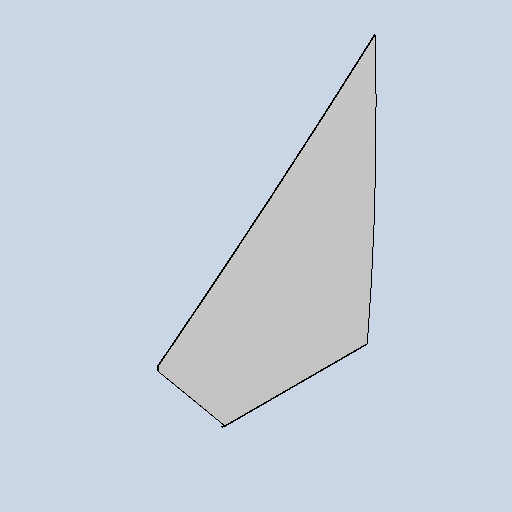
# Autodesk Inventor part: MSC 311 sheet left board face
Saved by Autodesk Inventor 2025 (Build 290162010, 162A)
## iProperties
Created: 2024-04-18
Part Number: MSC 311 sheet left board face
Material: AISI304
Document SubType Name: Sheet Metal
Designer: admin
Stock Number: МОО 311 лист левый борт морда
Mass: 48027.3 g
Surface Area: 40202.8 cm^2
Volume: 6003.41 cm^3
Density: 8 g/cm^3
Sheet Metal Rule: Default_mm
Sheet Metal Width: 980,000 mm
Sheet Metal Length: 1340,712 mm
Sheet Metal Area: 1313897,739 mm^2
Appearance: Default
Flat Pattern Width: 98 cm
Flat Pattern Length: 134.071 cm
Flat Pattern Area: 13139 cm^2
Author: admin
Autodesk Inventor part; units mm, degrees
ref_plane "YZ Plane" through (0, 0, 0) normal (1, 0, 0) x (0, 1, 0)
ref_plane "XZ Plane" through (0, 0, 0) normal (0, 1, 0) x (-1, 0, 0)
ref_plane "XY Plane" through (0, 0, 0) normal (0, 0, 1) x (1, 0, 0)
sketch "Sketch1" plane through (0, 0, 0) normal (0, 0, 1) x (1, 0, 0)
  line L0 (394.757121, -1035.809004) -> (394.757121, -1085.809004) construction
  line L1 (0, -1088.809004) -> (0, -1880) construction
  arc A0 (0.159434, -1878.130723) -> (0, 0) centre (-11009.945504, -940) ccw
  arc A1 (0, -1880) -> (0.159434, -1878.130723) centre (-11009.945504, -940) ccw construction
  arc A2 (-1.349222, -1881.302929) -> (0.159434, -1878.130723) centre (-4.822514, -1877.70623) ccw
  line L2 (-1.349222, -1881.302929) -> (0, -1880) construction
  line L3 (-71.93398, -1949.465837) -> (-1.349222, -1881.302929)
  line L4 (-247.746289, -1767.406862) -> (-71.93398, -1949.465837) construction
  line L5 (0, -1880) -> (0, 0) construction
  line L6 (0, -1880) -> (1.875639, -1880) construction
  dimension "d153" = 5
  dimension "d154" = 100
  dimension "d155" = 11050
  dimension "d156" = 136
  dimension "d157" = 1880
  measures "d153" radius of A2
  measures "d154" distance of L1.end L3.start
  measures "d155" radius of A0
  measures "d156" angle of L2 L6
  measures "d157" distance of L1.end L5.end
contour flange "Contour Flange2" sketch "Sketch1" thickness 3 bend radius 3 width 980 along (0, 0, 1) mid plane no both sides no wall seen from (-36.641601, -1915.384383, 0) lies toward (0.6946584, -0.7193398, 0) curves L3 A2 A0
bend "Bend2"
corner "Corner2"
sketch "Sketch2" plane through (0, 0, 0) normal (1, 0, 0) x (0, 1, 0)
  line L0 (-1878.385419, 980) -> (-1878.385419, 0)
  line L1 (-1878.385419, 0) -> (0.255204, 0)
  line L2 (0.255204, 0) -> (0.255204, 980)
  line L3 (-1878.385419, 980) -> (0.255204, 980)
  line L4 (-1883.460948, 980) -> (-1883.460948, 0)
  line L5 (-1951.623856, 980) -> (-1883.460948, 980)
  line L6 (-1951.623856, 0) -> (-1951.623856, 980)
  line L7 (-1951.623856, 0) -> (-1883.460948, 0)
  line L8 (-1878.385419, 980) -> (-1883.460948, 980)
  line L9 (-1878.385419, 0) -> (-1883.460948, 0)
  line L10 (-641.394796, 0) -> (-1463.712435, 980)
  line L11 (-1484.906708, 980) -> (-1951.623856, 588.377813)
  line L12 (-641.394796, 980) -> (-1463.712435, 0)
  line L13 (-1951.623856, 391.622187) -> (-1484.906708, 0)
  point P0 (0, 0)
  dimension "d160" = 300
  dimension "d162" = 40
  dimension "d163" = 40
  dimension "d164" = 40
  dimension "d172" = 641.65
  dimension "d173" = 641.65
  constraints: 12 end point, 8 point on line, 2 perpendicular, 1 collinear, 1 equal length
  measures "d160" distance from line of L11 L5.start
  measures "d162" angle of L3 L11
  measures "d163" angle of L2 L10
  measures "d164" angle of L2 L12
  measures "d172" distance of L10.start L1.end
  measures "d173" distance of L12.start L2.end
extrude "Extrusion2" cut sketch "Sketch2" along normal through all both and the other way through all contours L3 L11 L0 | L0 L11 L4 L8 | L4 L11 L6 L5 | L3 L12 L10 | L3 L2 L1 L10 L12
sketch "Sketch6" plane through (-1.349222, -1881.302929, 647.384078) normal (-0.6946584, 0.7193398, 0) x (0.7193398, 0.6946584, 0)
  line L0 (-77.68178, 471.026487) -> (-77.68178, 640.420835) construction
  line L1 (-77.68178, 640.420835) -> (-63.164852, 640.420835) construction
  line L2 (-63.164852, 640.420835) -> (-63.164852, 471.026487) construction
  line L3 (-63.164852, 471.026487) -> (-77.68178, 471.026487) construction
  point P0 (1307.833376, 647.384078)
  constraints: 2 other
mark "Mark4"
equation "\"d36\" = Thickness"
equation "\"d37\" = BendReliefWidth"
equation "\"d38\" = BendReliefDepth"
equation "\"d39\" = MinimumRemnant"
equation "\"d40\" = TransitionRadius"
equation "\"d42\" = BendRadius"
equation "\"d44\" = CornerReliefSize"
equation "\"d45\" = GapSize"
equation "\"d46\" = JacobiRadiusSize"
equation "\"BendRadius\" = Thickness"
equation "\"BendReliefWidth\" = Thickness"
equation "\"BendReliefDepth\" = 0.5 * Thickness"
equation "\"CornerReliefSize\" = 4 * Thickness"
equation "\"MinimumRemnant\" = 2 * Thickness"
equation "\"TransitionRadius\" = BendRadius"
equation "\"JacobiRadiusSize\" = BendRadius"
equation "\"GapSize\" = Thickness"
equation "\"Thickness\" = 3"
body "Solid3"
